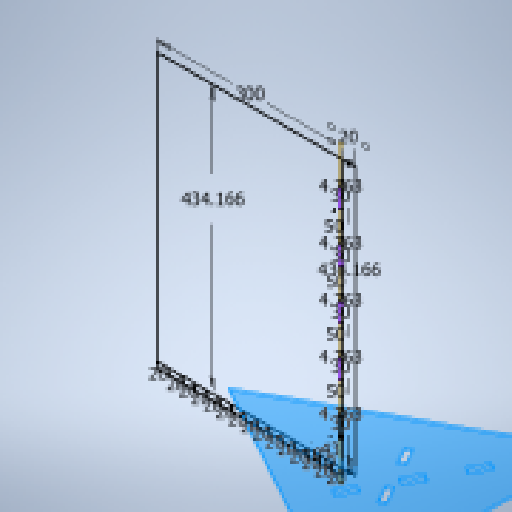
# Autodesk Inventor part: left back
Saved by Autodesk Inventor 2023 (Build 270158000, 158)
## iProperties
Created: 2023-09-18
Part Number: left back
Material: Polystyrene
Document SubType Name: Modeling
Designer: Nate
Density: 1.021 g/cm^3
Appearance: Smooth - White
Mass: 678.898 g
Surface Area: 2887.43 cm^2
Volume: 664.934 cm^3
Author: Nate
Autodesk Inventor part; units mm, degrees
ref_plane "YZ Plane" through (0, 0, 0) normal (1, 0, 0) x (0, 1, 0)
ref_plane "XZ Plane" through (0, 0, 0) normal (0, 1, 0) x (-1, 0, 0)
ref_plane "XY Plane" through (0, 0, 0) normal (0, 0, 1) x (1, 0, 0)
ref_plane "Work Plane1" through (0, 0, 0) normal (0, 0, 1) x (1, 0, 0)
sketch "Sketch1" plane through (0, 0, 0) normal (0, 0, 1) x (1, 0, 0)
  line L0 (0, 0) -> (-300, 0)
  line L1 (-300, 0) -> (-300, 434.166)
  line L2 (-300, 434.166) -> (0, 434.166)
  line L3 (0, 434.166) -> (0, 0)
  line L4 (0, 0) -> (20, 0)
  line L5 (20, 0) -> (20, 434.166)
  line L6 (20, 434.166) -> (0, 434.166)
  line L7 (0, 434.166) -> (0, 0)
  line L8 (0, 43) -> (-4.7625, 43)
  line L9 (-4.7625, 43) -> (-4.7625, 73)
  line L10 (-4.7625, 73) -> (0, 73)
  line L11 (0, 73) -> (0, 43)
  line L12 (0, 123) -> (-4.7625, 123)
  line L13 (-4.7625, 123) -> (-4.7625, 153)
  line L14 (-4.7625, 153) -> (0, 153)
  line L15 (0, 153) -> (0, 123)
  line L16 (0, 203) -> (-4.7625, 203)
  line L17 (-4.7625, 203) -> (-4.7625, 233)
  line L18 (-4.7625, 233) -> (0, 233)
  line L19 (0, 233) -> (0, 203)
  line L20 (0, 283) -> (-4.7625, 283)
  line L21 (-4.7625, 283) -> (-4.7625, 313)
  line L22 (-4.7625, 313) -> (0, 313)
  line L23 (0, 313) -> (0, 283)
  line L24 (0, 363) -> (-4.7625, 363)
  line L25 (-4.7625, 363) -> (-4.7625, 393)
  line L26 (-4.7625, 393) -> (0, 393)
  line L27 (0, 393) -> (0, 363)
  line L28 (0, 0) -> (-20, 0)
  line L29 (-20, 0) -> (-20, -10)
  line L30 (-20, -10) -> (0, -10)
  line L31 (0, -10) -> (0, 0)
  line L32 (-20, 0) -> (-40, 0)
  line L33 (-40, 0) -> (-40, -10)
  line L34 (-40, -10) -> (-20, -10)
  line L35 (-20, -10) -> (-20, 0)
  line L36 (-40, 0) -> (-60, 0)
  line L37 (-60, 0) -> (-60, -10)
  line L38 (-60, -10) -> (-40, -10)
  line L39 (-40, -10) -> (-40, 0)
  line L40 (-60, 0) -> (-80, 0)
  line L41 (-80, 0) -> (-80, -10)
  line L42 (-80, -10) -> (-60, -10)
  line L43 (-60, -10) -> (-60, 0)
  line L44 (-80, 0) -> (-100, 0)
  line L45 (-100, 0) -> (-100, -10)
  line L46 (-100, -10) -> (-80, -10)
  line L47 (-80, -10) -> (-80, 0)
  line L48 (-100, 0) -> (-120, 0)
  line L49 (-120, 0) -> (-120, -10)
  line L50 (-120, -10) -> (-100, -10)
  line L51 (-100, -10) -> (-100, 0)
  line L52 (-120, 0) -> (-140, 0)
  line L53 (-140, 0) -> (-140, -10)
  line L54 (-140, -10) -> (-120, -10)
  line L55 (-120, -10) -> (-120, 0)
  line L56 (-140, 0) -> (-160, 0)
  line L57 (-160, 0) -> (-160, -10)
  line L58 (-160, -10) -> (-140, -10)
  line L59 (-140, -10) -> (-140, 0)
  line L60 (-160, 0) -> (-180, 0)
  line L61 (-180, 0) -> (-180, -10)
  line L62 (-180, -10) -> (-160, -10)
  line L63 (-160, -10) -> (-160, 0)
  line L64 (-180, 0) -> (-200, 0)
  line L65 (-200, 0) -> (-200, -10)
  line L66 (-200, -10) -> (-180, -10)
  line L67 (-180, -10) -> (-180, 0)
  line L68 (-200, 0) -> (-220, 0)
  line L69 (-220, 0) -> (-220, -10)
  line L70 (-220, -10) -> (-200, -10)
  line L71 (-200, -10) -> (-200, 0)
  line L72 (-220, 0) -> (-240, 0)
  line L73 (-240, 0) -> (-240, -10)
  line L74 (-240, -10) -> (-220, -10)
  line L75 (-220, -10) -> (-220, 0)
  line L76 (-240, 0) -> (-260, 0)
  line L77 (-260, 0) -> (-260, -10)
  line L78 (-260, -10) -> (-240, -10)
  line L79 (-240, -10) -> (-240, 0)
  line L80 (-260, 0) -> (-280, 0)
  line L81 (-280, 0) -> (-280, -10)
  line L82 (-280, -10) -> (-260, -10)
  line L83 (-260, -10) -> (-260, 0)
  line L84 (-280, 0) -> (-300, 0)
  line L85 (-300, 0) -> (-300, -10)
  line L86 (-300, -10) -> (-280, -10)
  line L87 (-280, -10) -> (-280, 0)
  point P0 (10, 434.166)
  point P1 (10, 0)
  point P2 (-2.3813, 43)
  point P3 (0, 73)
  dimension "d0" = 300
  dimension "d2" = 434.166
  dimension "d3" = 20
  dimension "d4" = 434.166
  dimension "d5" = 4.7625
  dimension "d6" = 30
  dimension "d8" = 4.7625
  dimension "d9" = 30
  dimension "d10" = 4.7625
  dimension "d16" = 4.7625
  dimension "d18" = 4.7625
  dimension "d19" = 30
  dimension "d22" = 50
  dimension "d23" = 50
  dimension "d24" = 50
  dimension "d25" = 50
  dimension "d28" = 43
  dimension "d30" = 30
  dimension "d31" = 30
  dimension "d32" = 20
  dimension "d33" = 10
  dimension "d34" = 20
  dimension "d35" = 10
  dimension "d36" = 20
  dimension "d37" = 20
  dimension "d38" = 20
  dimension "d39" = 20
  dimension "d40" = 20
  dimension "d41" = 20
  dimension "d42" = 20
  dimension "d43" = 20
  dimension "d44" = 20
  dimension "d45" = 20
  dimension "d46" = 20
  dimension "d47" = 20
  dimension "d48" = 20
  constraints: 176 end point, 45 parallel, 22 horizontal, 22 perpendicular, 13 point on line, 3 midpoint, 2 collinear
  measures "d0" distance of L1.end L2.end
  measures "d2" distance between parallel lines of L2 L0
  measures "d3" distance of L6.end L5.end
  measures "d4" distance of point (10, 434.166) point (10, 0)
  measures "d5" distance of L9.end L10.end
  measures "d6" distance between parallel lines of L10 L8
  measures "d8" distance of L13.end L15.start
  measures "d9" distance between parallel lines of L14 L12
  measures "d10" distance of L17.end L19.start
  measures "d16" distance of L21.end L23.start
  measures "d18" distance of L25.end L27.start
  measures "d19" distance between parallel lines of L26 L24
  measures "d22" distance between parallel lines of L12 L10
  measures "d23" distance between parallel lines of L16 L14
  measures "d24" distance between parallel lines of L20 L18
  measures "d25" distance between parallel lines of L24 L22
  measures "d28" distance between parallel lines of L0 L8
  measures "d30" distance between parallel lines of L18 L16
  measures "d31" distance between parallel lines of L22 L20
  measures "d32" distance of L30.end L29.end
  measures "d33" distance of L29.end L28.end
  measures "d34" distance of L34.end L33.end
  measures "d35" distance of L33.end L32.end
  measures "d36" distance of L38.end L37.end
  measures "d37" distance of L42.end L41.end
  measures "d38" distance of L46.end L45.end
  measures "d39" distance of L50.end L49.end
  measures "d40" distance of L54.end L53.end
  measures "d41" distance of L58.end L57.end
  measures "d42" distance of L62.end L61.end
  measures "d43" distance of L66.end L65.end
  measures "d44" distance of L70.end L69.end
  measures "d45" distance of L74.end L73.end
  measures "d46" distance of L78.end L77.end
  measures "d47" distance of L82.end L81.end
  measures "d48" distance between parallel lines of L85 L81
extrude "Extrusion1" add sketch "Sketch1" along normal blind 4.7625 contours L0 L1 L2 L3 L26 L25 L24 L22 L21 L20 L18 L17 L16 L14 L13 L12 L10 L9 L8 | L3 L6 L5 L4 | L29 L34 L33 L0 | L37 L42 L41 L0 | L45 L50 L49 L0 | L0 L77 L82 L81 | L53 L58 L57 L0 | L0 L69 L74 L73 | L61 L66 L65 L0
body "Solid1"
